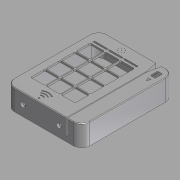
# Autodesk Inventor part: body
Saved by Autodesk Inventor 2014 SP2 (Build 180246200, 246)
## iProperties
Created: 2016-01-20
Part Number: body
Material: ABS plast
Document SubType Name: Modeling
Designer: Mervart
Mass: 39.7282 g
Surface Area: 400.615 cm^2
Volume: 37.4795 cm^3
Density: 1.06 g/cm^3
Appearance: 1.4571
LastSaveDate: 21.09.2010
Hmotnost: 0
Author: Mervart
Autodesk Inventor part; units mm, degrees
ref_plane "YZ Plane" through (0, 0, 0) normal (1, 0, 0) x (0, 1, 0)
ref_plane "XZ Plane" through (0, 0, 0) normal (0, 1, 0) x (-1, 0, 0)
ref_plane "XY Plane" through (0, 0, 0) normal (0, 0, 1) x (1, 0, 0)
sketch "Náčrt4" plane through (0, 0, 0) normal (0, 0, 1) x (1, 0, 0)
  line L0 (-45, -55) -> (45, -55)
  line L1 (45, -55) -> (45, 55)
  line L2 (45, 55) -> (-45, 55)
  line L3 (-45, 55) -> (-45, -55)
  line L4 (-45, -55) -> (45, 55) construction
  line L5 (45, -55) -> (-45, 55) construction
  point P0 (0, 0)
  dimension "d0" = 90
  dimension "d1" = 110
  constraints: 12 end point, 2 midpoint, 2 parallel, 1 horizontal, 1 perpendicular
  measures "d0" distance of L2.end L1.end
  measures "d1" distance of L1.end L0.end
extrude "Vysunutí1" add sketch "Náčrt4" along normal blind 25
fillet "Zaoblení1" radius 10 4 edges at (-45, 55, 12.5) (45, 55, 12.5) (45, -55, 12.5) (-45, -55, 12.5)
sketch "Náčrt5" plane through (0, 0, 25) normal (0, 0, 1) x (1, 0, 0)
  arc A0 (-45, -45) -> (-35, -55) centre (-35, -45) ccw construction
  line L0 (-35, -55) -> (35, -55) construction
  arc A1 (35, -55) -> (45, -45) centre (35, -45) ccw construction
  line L1 (45, -45) -> (45, 45) construction
  arc A2 (45, 45) -> (35, 55) centre (35, 45) ccw construction
  line L2 (35, 55) -> (-35, 55) construction
  arc A3 (-35, 55) -> (-45, 45) centre (-35, 45) ccw construction
  line L3 (-45, 45) -> (-45, -45) construction
  line L4 (27, 55) -> (27, -55)
  line L5 (28, 55) -> (28, -55)
  line L6 (27, -55) -> (28, -55)
  line L7 (27, 55) -> (28, 55)
  point P0 (0, 0)
  dimension "d5" = 1
  dimension "d6" = 72
  constraints: 8 end point, 4 point on line, 2 collinear, 2 perpendicular
  measures "d5" distance between parallel lines of L5 L4
  measures "d6" distance between parallel lines of L3 L4
extrude "Vysunutí2" cut sketch "Náčrt5" against normal blind 19
sketch "Náčrt6" plane through (0, 0, 25) normal (0, 0, 1) x (1, 0, 0)
  line L0 (27, -55) -> (27, 55) construction
  line L1 (27, 55) -> (-35, 55) construction
  arc A0 (-35, 55) -> (-45, 45) centre (-35, 45) ccw construction
  line L2 (-45, 45) -> (-45, -45) construction
  arc A1 (-45, -45) -> (-35, -55) centre (-35, -45) ccw construction
  line L3 (-35, -55) -> (27, -55) construction
  line L4 (28, 55) -> (28, -55) construction
  line L5 (28, -55) -> (35, -55) construction
  arc A2 (35, -55) -> (45, -45) centre (35, -45) ccw construction
  line L6 (45, -45) -> (45, 45) construction
  arc A3 (45, 45) -> (35, 55) centre (35, 45) ccw construction
  line L7 (35, 55) -> (28, 55) construction
  line L8 (27, -55) -> (27, 55) construction
  line L9 (28, -55) -> (27, -55) construction
  line L10 (28, 55) -> (28, -55) construction
  line L11 (27, 55) -> (28, 55) construction
  line L12 (27, 55) -> (24, 55)
  line L13 (24, 55) -> (27, 40)
  line L14 (27, 55) -> (27, 40)
  line L15 (28, 55) -> (31, 55)
  line L16 (28, 55) -> (28, 40)
  line L17 (28, 40) -> (31, 55)
  point P0 (0, 0)
  dimension "d9" = 3
  dimension "d10" = 15
  dimension "d11" = 3
  dimension "d12" = 15
  constraints: 12 end point, 4 point on line
  measures "d9" distance of L8.end L12.end
  measures "d10" distance of L13.end L8.end
  measures "d11" distance of L10.start L15.end
  measures "d12" distance of L10.start L16.end
extrude "Vysunutí3" cut sketch "Náčrt6" against normal blind 19
sketch "Náčrt7" plane through (0, 0, 25) normal (0, 0, 1) x (1, 0, 0)
  line L0 (-36, 36.3) -> (-19, 36.3)
  line L1 (-19, 36.3) -> (-19, 19.3)
  line L2 (-19, 19.3) -> (-36, 19.3)
  line L3 (-36, 19.3) -> (-36, 36.3)
  line L4 (-36, 36.3) -> (-19, 19.3) construction
  line L5 (-19, 36.3) -> (-36, 19.3) construction
  line L6 (27, 40) -> (24, 55) construction
  line L7 (24, 55) -> (-35, 55) construction
  arc A0 (-35, 55) -> (-45, 45) centre (-35, 45) ccw construction
  line L8 (-45, 45) -> (-45, -45) construction
  arc A1 (-45, -45) -> (-35, -55) centre (-35, -45) ccw construction
  line L9 (-35, -55) -> (27, -55) construction
  line L10 (27, -55) -> (27, 40) construction
  line L11 (-18, 36.3) -> (-1, 36.3) construction
  line L12 (-1, 36.3) -> (-1, 19.3) construction
  line L13 (-1, 19.3) -> (-18, 19.3) construction
  line L14 (-18, 19.3) -> (-18, 36.3) construction
  line L15 (0, 36.3) -> (17, 36.3) construction
  line L16 (17, 36.3) -> (17, 19.3) construction
  line L17 (17, 19.3) -> (0, 19.3) construction
  line L18 (0, 19.3) -> (0, 36.3) construction
  line L19 (-36, 18.3) -> (-19, 18.3) construction
  line L20 (-19, 18.3) -> (-19, 1.3) construction
  line L21 (-19, 1.3) -> (-36, 1.3) construction
  line L22 (-36, 1.3) -> (-36, 18.3) construction
  line L23 (-18, 18.3) -> (-1, 18.3) construction
  line L24 (-1, 18.3) -> (-1, 1.3) construction
  line L25 (-1, 1.3) -> (-18, 1.3) construction
  line L26 (-18, 1.3) -> (-18, 18.3) construction
  line L27 (0, 18.3) -> (17, 18.3) construction
  line L28 (17, 18.3) -> (17, 1.3) construction
  line L29 (17, 1.3) -> (0, 1.3) construction
  line L30 (0, 1.3) -> (0, 18.3) construction
  line L31 (-36, 0.3) -> (-19, 0.3) construction
  line L32 (-19, 0.3) -> (-19, -16.7) construction
  line L33 (-19, -16.7) -> (-36, -16.7) construction
  line L34 (-36, -16.7) -> (-36, 0.3) construction
  line L35 (-18, 0.3) -> (-1, 0.3) construction
  line L36 (-1, 0.3) -> (-1, -16.7) construction
  line L37 (-1, -16.7) -> (-18, -16.7) construction
  line L38 (-18, -16.7) -> (-18, 0.3) construction
  line L39 (0, 0.3) -> (17, 0.3) construction
  line L40 (17, 0.3) -> (17, -16.7) construction
  line L41 (17, -16.7) -> (0, -16.7) construction
  line L42 (0, -16.7) -> (0, 0.3) construction
  line L43 (-36, -17.7) -> (-19, -17.7) construction
  line L44 (-19, -17.7) -> (-19, -34.7) construction
  line L45 (-19, -34.7) -> (-36, -34.7) construction
  line L46 (-36, -34.7) -> (-36, -17.7) construction
  line L47 (-18, -17.7) -> (-1, -17.7) construction
  line L48 (-1, -17.7) -> (-1, -34.7) construction
  line L49 (-1, -34.7) -> (-18, -34.7) construction
  line L50 (-18, -34.7) -> (-18, -17.7) construction
  line L51 (0, -17.7) -> (17, -17.7) construction
  line L52 (17, -17.7) -> (17, -34.7) construction
  line L53 (17, -34.7) -> (0, -34.7) construction
  line L54 (0, -34.7) -> (0, -17.7) construction
  point P0 (0, 0)
  point P1 (-27.5, 27.8)
  dimension "d16" = 17
  dimension "d17" = 17
  dimension "d18" = 18.7
  dimension "d19" = 9
  dimension "d22" = 18
  dimension "d25" = 18
  dimension "d28" = 10
  dimension "d29" = 20.3
  constraints: 100 end point, 2 collinear, 2 horizontal, 2 midpoint, 2 parallel, 1 perpendicular, 1 vertical, 86 other
  measures "d16" distance of L1.end L2.end
  measures "d17" distance of L0.end L1.end
  measures "d18" distance between parallel lines of L7 L0
  measures "d19" distance between parallel lines of L8 L3
  measures "d22" distance of L0.end L12.start
  measures "d25" distance of L0.end L20.start
  measures "d28" distance between parallel lines of L10 L28
  measures "d29" distance between parallel lines of L9 L49
shell "Skořepina1" thickness 2 removed faces 1 at (-15, 15, 0)
extrude "Vysunutí4" cut sketch "Náčrt7" against normal blind 19
sketch "Náčrt8" plane through (0, 0, 25) normal (0, 0, 1) x (1, 0, 0)
  line L0 (27, 40) -> (24, 55) construction
  line L1 (24, 55) -> (-35, 55) construction
  arc A0 (-35, 55) -> (-45, 45) centre (-35, 45) ccw construction
  line L2 (-45, 45) -> (-45, -45) construction
  arc A1 (-45, -45) -> (-35, -55) centre (-35, -45) ccw construction
  line L3 (-35, -55) -> (27, -55) construction
  line L4 (27, -55) -> (27, 40) construction
  line L5 (-9.5, 36.3) -> (-9.5, 55) construction
  circle A2 centre (-9.49, 47) radius 7 construction
  circle A3 centre (-9.49, 47) radius 5 construction
  circle A4 centre (-9.49, 47) radius 3.5 construction
  line L6 (-9.49, 47) -> (5.8677, 47) construction
  line L7 (-9.49, 47) -> (-19.8655, 57.3755) construction
  line L8 (-9.49, 47) -> (5.1832, 47) construction
  line L9 (-9.49, 47) -> (-23.0462, 52.6152) construction
  line L10 (-9.49, 47) -> (-24.1631, 47) construction
  line L11 (-9.49, 47) -> (-23.0462, 41.3848) construction
  line L12 (-9.49, 47) -> (-19.8655, 36.6245) construction
  line L13 (-9.49, 47) -> (-15.1051, 33.4438) construction
  line L14 (-9.49, 47) -> (-9.49, 32.3268) construction
  line L15 (-9.49, 47) -> (-3.8748, 33.4438) construction
  line L16 (-9.49, 47) -> (0.8855, 36.6245) construction
  line L17 (-9.49, 47) -> (4.0663, 41.3848) construction
  line L18 (-9.49, 47) -> (5.1832, 47) construction
  line L19 (-9.49, 47) -> (4.0663, 52.6152) construction
  line L20 (-9.49, 47) -> (0.8855, 57.3755) construction
  line L21 (-9.49, 47) -> (-3.8748, 60.5562) construction
  line L22 (-9.49, 47) -> (-9.49, 61.6732) construction
  line L23 (-9.49, 47) -> (-15.1051, 60.5562) construction
  point P0 (0, 0)
  point P1 (-16.49, 47)
  point P2 (-9.49, 54)
  point P3 (-2.49, 47)
  point P4 (-9.49, 40)
  point P5 (-14.4397, 51.9497)
  point P6 (-4.5402, 51.9497)
  point P7 (-4.5402, 42.0503)
  point P8 (-14.4397, 42.0503)
  point P9 (-14.1094, 48.9134)
  point P10 (-14.1094, 45.0866)
  point P11 (-11.4034, 42.3806)
  point P12 (-7.5766, 42.3806)
  point P13 (-4.8706, 45.0866)
  point P14 (-4.8706, 48.9134)
  point P15 (-7.5766, 51.6194)
  point P16 (-11.4034, 51.6194)
  point P17 (-11.9648, 49.4749)
  point P18 (-12.99, 47)
  point P19 (-11.9648, 44.5251)
  point P20 (-9.49, 43.5)
  point P21 (-7.0151, 44.5251)
  point P22 (-5.99, 47)
  point P23 (-7.0151, 49.4749)
  point P24 (-9.49, 50.5)
  point P25 (-12.7235, 48.3394)
  point P26 (-10.8294, 50.2336)
  point P27 (-8.1506, 50.2336)
  point P28 (-6.2564, 48.3394)
  point P29 (-6.2564, 45.6606)
  point P30 (-8.1506, 43.7664)
  point P31 (-10.8294, 43.7664)
  point P32 (-12.7235, 45.6606)
  dimension "d35" = 14
  dimension "d36" = 10
  dimension "d37" = 7
  dimension "d33" = 72
  dimension "d38" = 135
  dimension "d41" = 360
  dimension "d94" = 8
  constraints: 38 end point, 29 point on line, 5 coincident, 1 equal length, 1 horizontal, 85 other
  measures "d33" distance between parallel lines of L4 L2
  measures "d38" angle of L8 L7
  measures "d94" distance from line of L1 point (-9.49, 47)
hole "Díra1" at (-9.49, 47, 25) at (-11.9648, 49.4749, 25) at (-12.99, 47, 25) at (-11.9648, 44.5251, 25) at (-9.49, 43.5, 25) at (-7.0151, 44.5251, 25) at (-5.99, 47, 25) at (-7.0151, 49.4749, 25) at (-9.49, 50.5, 25) direction (0, 0, -1) diameter 0.6 end through all
chamfer "Zkosení1" distance 0.7 angle 45 13 edges at (-5.5, 55, 25) (-42.0711, 52.0711, 25) (-45, 0, 25) (-42.0711, -52.0711, 25) (-4, -55, 25) (24, 55, 15.5) (27.5, 55, 6) (31, 55, 15.5) (42.0711, 52.0711, 25) (45, 0, 25) (42.0711, -52.0711, 25) (31.5, -55, 25) (33, 55, 25)
sketch "Náčrt9" plane through (0, 0, 25) normal (0, 0, 1) x (1, 0, 0)
  line L0 (-35, 54.3) -> (24.14, 54.3) construction
  arc A0 (-35, 54.3) -> (-44.3, 45) centre (-35, 45) ccw construction
  line L1 (-44.3, -45) -> (-44.3, 45) construction
  arc A1 (-44.3, -45) -> (-35, -54.3) centre (-35, -45) ccw construction
  line L2 (27, -54.3) -> (-35, -54.3) construction
  line L3 (27, -54.3) -> (27, 40) construction
  line L4 (27, 40) -> (24.14, 54.3) construction
  circle A2 centre (-9.49, 50.5) radius 0.3 construction
  circle A3 centre (-5.99, 47) radius 0.3 construction
  circle A4 centre (-9.49, 43.5) radius 0.3 construction
  circle A5 centre (-12.99, 47) radius 0.3 construction
  circle A6 centre (-9.49, 47) radius 0.3 construction
  circle A7 centre (-11.9648, 49.4749) radius 0.3 construction
  circle A8 centre (-11.9648, 44.5251) radius 0.3 construction
  circle A9 centre (-7.0151, 44.5251) radius 0.3 construction
  circle A10 centre (-7.0151, 49.4749) radius 0.3 construction
  line L5 (-35, 40.8) -> (-20, 40.8)
  line L6 (-19, 39.8) -> (-19, 39.8)
  line L7 (-20, 38.8) -> (-35, 38.8)
  line L8 (-36, 39.8) -> (-36, 39.8)
  line L9 (-19, 36.3) -> (-36, 36.3) projected
  arc A11 (-35, 40.8) -> (-36, 39.8) centre (-35, 39.8) ccw
  arc A12 (-36, 39.8) -> (-35, 38.8) centre (-35, 39.8) ccw
  arc A13 (-19, 39.8) -> (-20, 40.8) centre (-20, 39.8) ccw
  arc A14 (-20, 38.8) -> (-19, 39.8) centre (-20, 39.8) ccw
  point P0 (0, 0)
  point P1 (-36, 40.8)
  point P2 (-19, 38.8)
  point P3 (-19, 40.8)
  point P4 (-36, 38.8)
  dimension "d55" = 17
  dimension "d59" = 2
  dimension "d122" = 2.5
  dimension "d123" = 1
  constraints: 8 end point, 8 point on circle, 8 point on line, 8 tangent, 4 centre point, 3 equal radius, 2 parallel, 1 horizontal, 1 perpendicular
  measures "d55" distance of L9.end L9.start
  measures "d59" distance between parallel lines of L7 L5
  measures "d122" distance between parallel lines of L9 L7
  measures "d123" radius of A11
extrude "Vysunutí5" cut sketch "Náčrt9" against normal blind 10
pattern_linear "Obdélníkové pole1" count 3 spacing 18 along (1, 0, 0) of "Vysunutí5"
sketch "Náčrt10" plane through (-35, -55, 0) normal (0, -1, 0) x (1, 0, 0)
  line L0 (63, 24.3) -> (70, 24.3) construction
  line L1 (63, 24.3) -> (63, 6) construction
  line L2 (63, 6) -> (62, 6) construction
  line L3 (62, 6) -> (62, 24.3) construction
  line L4 (0, 24.3) -> (62, 24.3) construction
  line L5 (0, 0) -> (0, 24.3) construction
  line L6 (0, 0) -> (70, 0) construction
  line L7 (70, 24.3) -> (70, 0) construction
  line L8 (4.1149, 12.5) -> (57.5383, 12.5) construction
  point P0 (35, 0)
  point P1 (10, 12.5)
  point P2 (53, 12.5)
  dimension "d65" = 12.5
  dimension "d66" = 10
  dimension "d67" = 43
  constraints: 2 end point, 2 point on line, 1 perpendicular
  measures "d65" distance between parallel lines of L6 L8
  measures "d66" distance from line of L5 point (10, 12.5)
  measures "d67" distance of point (53, 12.5) point (10, 12.5)
hole "Díra2" at (-25, -55, 12.5) at (18, -55, 12.5) direction (0, 1, 0) diameter 3.1 depth 2 tip angle 118 countersink diameter 6.3 countersink angle 90
sketch "Náčrt11" plane through (0, 0, 25) normal (0, 0, 1) x (1, 0, 0)
  line L0 (33.3, 47.3) -> (39.3, 47.3)
  line L1 (39.3, 47.3) -> (39.3, 38.3)
  line L2 (39.3, 38.3) -> (33.3, 38.3)
  line L3 (33.3, 38.3) -> (33.3, 47.3)
  line L4 (44.3, 45) -> (44.3, -45) projected
  line L5 (30.86, 54.3) -> (35, 54.3) projected
  line L6 (35, 47.3) -> (35, 38.3)
  line L7 (35.5, 47.3) -> (35.5, 38.3)
  line L8 (34.3, 34.7626) -> (38.3, 34.7626)
  line L9 (38.3, 34.7626) -> (36.3, 30.7626)
  line L10 (36.3, 30.7626) -> (34.3, 34.7626)
  point P0 (0, 0)
  point P1 (36.3, 34.7626)
  dimension "d76" = 6
  dimension "d77" = 9
  dimension "d78" = 5
  dimension "d79" = 7
  dimension "d84" = 1.7
  dimension "d85" = 0.5
  dimension "d89" = 4
  dimension "d90" = 1
  dimension "d91" = 4
  constraints: 18 end point, 4 perpendicular, 4 point on line, 2 parallel, 1 horizontal, 1 midpoint, 1 vertical alignment
  measures "d76" distance of L0.start L0.end
  measures "d77" distance of L2.end L0.start
  measures "d78" distance between parallel lines of L4 L1
  measures "d79" distance between parallel lines of L5 L0
  measures "d84" distance between parallel lines of L6 L3
  measures "d85" distance between parallel lines of L7 L6
  measures "d89" distance of L8.start L8.end
  measures "d90" horizontal distance of L8.start L2.end
  measures "d91" distance from line of L9.end L8
extrude "Vysunutí6" add sketch "Náčrt11" along normal blind 0.03 contours L0 L6 L2 L3 | L0 L1 L2 L7 | L8 L9 L10
fillet "Zaoblení3" radius 1 4 edges at (39.3, 38.3, 25.015) (39.3, 47.3, 25.015) (33.3, 47.3, 25.015) (33.3, 38.3, 25.015)
sketch "Náčrt12" plane through (0, 0, 25) normal (0, 0, 1) x (1, 0, 0)
  line L0 (-35, 40.8) -> (-20, 40.8) construction
  line L1 (-20, 38.8) -> (-35, 38.8) construction
  line L2 (-35, 54.3) -> (24.14, 54.3) construction
  arc A0 (-35, 54.3) -> (-44.3, 45) centre (-35, 45) ccw construction
  line L3 (-44.3, -45) -> (-44.3, 45) construction
  arc A1 (-44.3, -45) -> (-35, -54.3) centre (-35, -45) ccw construction
  line L4 (27, -54.3) -> (-35, -54.3) construction
  line L5 (27, -54.3) -> (27, 40) construction
  line L6 (27, 40) -> (24.14, 54.3) construction
  circle A2 centre (-9.49, 50.5) radius 0.3 construction
  circle A3 centre (-5.99, 47) radius 0.3 construction
  circle A4 centre (-9.49, 43.5) radius 0.3 construction
  circle A5 centre (-12.99, 47) radius 0.3 construction
  circle A6 centre (-9.49, 47) radius 0.3 construction
  circle A7 centre (-11.9648, 49.4749) radius 0.3 construction
  circle A8 centre (-11.9648, 44.5251) radius 0.3 construction
  circle A9 centre (-7.0151, 44.5251) radius 0.3 construction
  circle A10 centre (-7.0151, 49.4749) radius 0.3 construction
  line L7 (-9.5, -34.7) -> (-9.5, -59.9836) construction
  circle A11 centre (-9.5, -51.2094) radius 0.9
  line L8 (-9.5, -51.2094) -> (7.5045, -51.2094) construction
  line L9 (-9.5, -51.2094) -> (-9.95, -50.4299) construction
  line L10 (-9.5, -51.2094) -> (-9.05, -50.4299) construction
  arc A12 (-12.7708, -54.3) -> (-5, -51.2094) centre (-9.5, -51.2094) ccw construction
  arc A13 (-7.55, -47.8319) -> (-11.45, -47.8319) centre (-9.5, -51.2094) ccw
  arc A14 (-13.8056, -54.3) -> (-4.2, -51.2094) centre (-9.5, -51.2094) ccw construction
  arc A15 (-6.9764, -47.0127) -> (-12.0236, -47.0127) centre (-9.5, -51.2094) ccw
  arc A16 (-17.7394, -54.3) -> (-0.7, -51.2094) centre (-9.5, -51.2094) ccw construction
  arc A17 (-5.372, -45.314) -> (-13.628, -45.314) centre (-9.5, -51.2094) ccw
  arc A18 (-18.5889, -54.3) -> (0.1, -51.2094) centre (-9.5, -51.2094) ccw construction
  arc A19 (-4.7984, -44.4948) -> (-14.2016, -44.4948) centre (-9.5, -51.2094) ccw
  arc A20 (-22.2302, -54.3) -> (3.6, -51.2094) centre (-9.5, -51.2094) ccw construction
  arc A21 (-3.4792, -42.6108) -> (-15.5208, -42.6108) centre (-9.5, -51.2094) ccw
  arc A22 (-23.052, -54.3) -> (4.4, -51.2094) centre (-9.5, -51.2094) ccw construction
  arc A23 (-2.9056, -41.7916) -> (-16.0944, -41.7916) centre (-9.5, -51.2094) ccw
  line L11 (-7.55, -47.8319) -> (-6.9764, -47.0127)
  line L12 (-5.372, -45.314) -> (-4.7984, -44.4948)
  line L13 (-15.5208, -42.6108) -> (-16.0944, -41.7916)
  line L14 (-11.45, -47.8319) -> (-12.0236, -47.0127)
  line L15 (-13.628, -45.314) -> (-14.2016, -44.4948)
  line L16 (-3.4792, -42.6108) -> (-2.9056, -41.7916)
  line L17 (0.0317, -34.7) -> (5.0582, -25.9939) construction
  arc A24 (-35, 40.8) -> (-35, 38.8) centre (-35, 39.8) ccw projected
  arc A25 (-20, 38.8) -> (-20, 40.8) centre (-20, 39.8) ccw projected
  point P0 (0, 0)
  point P1 (-9.5, -44.0124)
  point P2 (-9.5, -40.7124)
  dimension "d96" = 1.8
  dimension "d109" = 3
  dimension "d110" = 1
  dimension "d111" = 1
  dimension "d112" = 1
  dimension "d113" = 2.3
  dimension "d114" = 2.3
  dimension "d115" = 35
  dimension "d116" = 35
  dimension "d117" = 35
  dimension "d119" = 35
  dimension "d120" = 35
  dimension "d121" = 35
  constraints: 28 point on circle, 22 end point, 13 centre point, 13 point on line, 6 coincident, 2 vertical alignment, 1 horizontal
  measures "d96" diameter of A11
  measures "d109" radial gap between concentric circles of A11 A13
  measures "d110" distance of L14.start L14.end
  measures "d111" distance of L15.start L15.end
  measures "d112" distance of L13.start L13.end
  measures "d113" radial gap between concentric circles of A17 A15
  measures "d114" radial gap between concentric circles of A21 A19
  measures "d115" angle of L7 L14
  measures "d116" angle of L7 L15
  measures "d117" angle of L7 L13
  measures "d119" angle of L11 L7
  measures "d120" angle of L12 L7
  measures "d121" angle of L16 L7
extrude "Vysunutí7" add sketch "Náčrt12" along normal blind 0.03
fillet "Zaoblení4" radius 1.5 4 edges at (-36, 36.3, 24) (-19, 36.3, 24) (-19, 19.3, 24) (-36, 19.3, 24)
pattern_linear "Obdélníkové pole2" count 3 spacing 18 along (1, 0, 0) count 4 spacing 18 along (0, -1, 0) of "Zaoblení4", "Vysunutí4"
equation "\"d11\" = d9"
equation "\"d12\" = d10"
equation "\"d16\" = d17"
